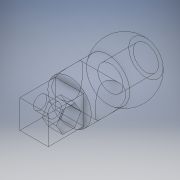
# Autodesk Inventor part: Now as three Part 2
Saved by Autodesk Inventor 2017 (Build 210142000, 142)
## iProperties
Created: 2017-04-12
Part Number: Now as three Part 2
Material: Generic
Document SubType Name: Modeling
Designer: andrew
Density: 1 g/cm^3
Appearance: Default
Author: andrew
Autodesk Inventor part; units mm, degrees
ref_plane "YZ Plane" through (0, 0, 0) normal (1, 0, 0) x (0, 1, 0)
ref_plane "XZ Plane" through (0, 0, 0) normal (0, 1, 0) x (-1, 0, 0)
ref_plane "XY Plane" through (0, 0, 0) normal (0, 0, 1) x (1, 0, 0)
sketch "Sketch1" plane through (0, 0, 0) normal (0, 0, 1) x (1, 0, 0)
  line L0 (0, 6.1628) -> (0, 4.6128)
  line L1 (0, 0) -> (0, -5.3285)
  line L2 (0, -7.6236) -> (0, 6.1628)
  line L3 (7.7918, 0) -> (42.6907, 0)
  line L4 (6.1094, -12.088) -> (6.1094, -4.669)
  line L5 (-6.1094, -10.2236) -> (-6.1094, -4.5067)
  line L6 (0, -7.6236) -> (0, -10.2236)
  line L7 (0, -7.6236) -> (0, -5.0236) construction
  arc A0 (-6.1094, 5.0092) -> (-6.87, -3.5101) centre (0, 0.1701) ccw
  arc A1 (6.1094, -4.669) -> (4.9829, 6.1628) centre (0, 0.1701) ccw
  circle A2 centre (27.3823, 0) radius 1.6
  circle A3 centre (27.3823, 0) radius 1.6
  arc A4 (15.7262, -19.2861) -> (15.9651, 19.4308) centre (0.0053, 0.1701) ccw
  arc A5 (14.9776, -18.1086) -> (14.9776, 18.1086) centre (0, 0) ccw construction
  line L8 (25.0186, 0.0157) -> (19.4598, 0.0157) construction
  line L9 (22.9824, -8.2534) -> (24.1975, 0.0157) construction
  line L10 (24.1975, 0.0157) -> (22.8643, 8.3172) construction
  line L11 (28.9823, 0) -> (30.9823, 0) construction
  line L12 (33.1204, -3.5101) -> (30.9986, 0.1649)
  line L13 (39.4857, -3.5101) -> (33.1204, -3.5101)
  line L14 (39.4857, 0.1649) -> (37.3639, -3.5101)
  circle A6 centre (35.2258, 0) radius 1.9
  line L15 (30.9986, 0.1649) -> (33.1239, 3.846)
  line L16 (33.1239, 3.846) -> (39.4857, 3.8504)
  line L17 (37.3639, 3.8489) -> (39.4857, 0.1649)
  line L18 (39.4857, 0.1784) -> (39.4857, 3.8504)
  line L19 (39.4857, 3.8504) -> (39.4857, -3.5101)
  line L20 (39.4857, 3.8504) -> (39.4857, 5.8504)
  line L21 (39.4857, 5.8504) -> (23.6696, 8.2698)
  arc A7 (15.7262, -19.2861) -> (15.9651, 19.4308) centre (0, 0.1701) ccw
  line L22 (39.4857, -3.5101) -> (39.4857, -5.5101)
  line L23 (39.4857, -5.5101) -> (23.6696, -7.9296)
  line L24 (23.6696, -7.9296) -> (23.6696, 8.2698)
  line L25 (0, 6.1628) -> (0, -10.2236)
  line L26 (0, -12.323) -> (0, -15.7561)
  line L27 (10.9155, -5.0236) -> (17.2808, -5.0236)
  line L28 (17.2808, -8.6986) -> (15.159, -12.3736)
  circle A8 centre (13.0373, -8.6986) radius 1.9
  line L29 (8.7937, -8.6986) -> (10.9155, -5.0236)
  line L30 (17.2808, -12.3736) -> (10.9155, -12.3736)
  line L31 (10.9155, -12.3736) -> (8.7937, -8.6986)
  line L32 (15.159, -5.0236) -> (17.2808, -8.6986)
  line L33 (10.9155, -12.3736) -> (10.9155, -14.3736)
  line L34 (-6.1094, -10.2236) -> (-6.1094, -14.3736)
  line L35 (0, -14.3736) -> (0, -10.2236)
  line L36 (0, -14.3736) -> (0, -19.3736)
  line L37 (-6.1094, -19.3736) -> (-6.1094, -14.3736)
  line L38 (0, -19.3736) -> (0, -25.3736)
  line L39 (0, -25.3736) -> (-6.1094, -25.3736)
  line L40 (-6.1094, -25.3736) -> (-6.1094, -19.3736)
  arc A9 (-4.8255, 6.1628) -> (-6.1094, -4.5067) centre (0, 0.1701) ccw
  line L41 (-5.029, 6.1628) -> (-4.9829, 6.1628)
  line L42 (-4.8255, 6.1628) -> (0, 6.1628)
  dimension "d2" = 3.8
  dimension "d3" = 2
  dimension "d4" = 2
  dimension "d5" = 16
  dimension "d6" = 2
  dimension "d7" = 16
  dimension "d9" = 3.8
  dimension "d10" = 2
  dimension "d17" = 5
  dimension "d50" = 6
  dimension "d64" = 7.7937
  dimension "d65" = 15.388
  constraints: 86 end point, 16 point on circle, 10 centre point, 10 point on line, 6 vertical, 2 collinear, 2 perpendicular, 1 coincident, 1 horizontal, 1 parallel
  measures "d2" diameter of A6
  measures "d3" distance of L11.start L11.end
  measures "d4" distance of L16.end L21.start
  measures "d5" distance of L21.start L21.end
  measures "d6" distance of L19.end L22.end
  measures "d7" distance of L22.end L23.end
  measures "d9" diameter of A8
  measures "d10" distance of L30.end L33.end
  measures "d17" distance of L35.start L36.end
  measures "d50" distance of L36.end L38.end
  measures "d64" radius of A0
  measures "d65" diameter of A9
revolve "Revolution1" add sketch "Sketch1" angle 360 about axis through (0, -12.323, 0) along (0, -1, 0) contours L0 L2 L1 L6 L35 L26 L36 L38 L39 L40 L37 L34 L5 A9 L42
sketch "Sketch2" plane through (0, 0, 0) normal (1, 0, 0) x (0, 1, 0)
  line L0 (-4.669, 0) -> (-6.7907, -3.675) construction
  line L1 (-6.7907, 3.675) -> (-4.669, 0) construction
  line L2 (-15.156, 0) -> (-13.156, 0) construction
  line L3 (-11.0343, -3.675) -> (-6.7907, -3.675) construction
  line L4 (-4.5067, -6.1094) -> (-4.5067, 6.1094) construction
  line L5 (-4.5067, -6.1094) -> (-4.5067, 6.1094) construction
  line L6 (-48.8073, 0) -> (-58.5119, 0) construction
  line L7 (-8.9125, 0) -> (-6.3144, -1.5) construction
  line L8 (-17.8945, -2.9836) -> (-21.3586, -2.9836)
  line L9 (-21.3586, -2.9836) -> (-23.0907, 0.0164)
  line L10 (-23.0907, 0.0164) -> (-21.3586, 3.0164)
  line L11 (-21.3586, 3.0164) -> (-17.8945, 3.0164)
  line L12 (-17.8945, 3.0164) -> (-16.1625, 0.0164)
  line L13 (-16.1625, 0.0164) -> (-17.8945, -2.9836)
  line L14 (23.6533, 6.6124) -> (23.3606, 8.9041) construction
  line L15 (29.9823, 11.5805) -> (34.9823, 11.5805) construction
  line L16 (24.1789, 0) -> (22.8458, 8.3015) construction
  line L17 (25, 0) -> (19.4412, 0) construction
  line L18 (25.1551, -0.0164) -> (29.5051, -0.0164) construction
  line L19 (23.6533, -6.0645) -> (23.6533, 6.6124) construction
  arc A0 (14.9776, -18.1086) -> (14.9776, 18.1086) centre (0, 0) ccw construction
  arc A1 (18.0021, -17.3472) -> (18.0021, 17.3472) centre (0, 0) ccw construction
  arc A2 (18.0021, -17.3472) -> (18.0021, 17.3472) centre (0, 0) ccw construction
  line L20 (22.9638, -8.2692) -> (24.1789, 0) construction
  circle A3 centre (29.5051, -0.0164) radius 4.35 construction
  line L21 (43.4694, -5.828) -> (23.3606, -8.9041) construction
  line L22 (43.4694, 5.828) -> (23.3606, 8.9041) construction
  line L23 (37.4871, -3) -> (35.7551, 0) construction
  line L24 (35.7551, 0) -> (37.4871, 3) construction
  line L25 (43.4694, 5.828) -> (43.4694, -5.828) construction
  circle A4 centre (39.2192, 0) radius 1.9 construction
  line L26 (25, 0) -> (20.4835, 0) construction
  line L27 (23.6533, -6.0645) -> (23.3606, -8.9041) construction
  line L28 (43.4694, 0) -> (43.4694, 5.828) construction
  line L29 (43.4694, -5.828) -> (43.4694, 5.828) construction
  line L30 (29.5346, 0.0703) -> (29.5346, 0.0867) construction
  line L31 (37.4871, 3) -> (43.4694, 3.5234) construction
  line L32 (37.4871, -3) -> (43.4694, -3.5234) construction
  circle A5 centre (-17.0481, 18.2856) radius 1.75
  line L33 (-15.4481, 18.2856) -> (-13.4481, 18.2856) construction
  line L34 (-11.3263, 14.6106) -> (-13.4481, 18.2856) construction
  line L35 (-13.4481, 18.2856) -> (-11.3263, 21.9606) construction
  circle A6 centre (-9.2045, 18.2856) radius 1.9
  line L36 (-4.961, 18.2856) -> (-7.0828, 14.6106) construction
  line L37 (-7.0828, 21.9606) -> (-4.961, 18.2856) construction
  line L38 (-11.3263, 21.9606) -> (-7.0828, 21.9606) construction
  line L39 (-11.3263, 14.6106) -> (-7.0828, 14.6106) construction
  line L40 (-9.2045, 18.2856) -> (-6.6065, 16.7856)
  line L41 (-7.4725, 15.2856) -> (-10.9366, 15.2856)
  line L42 (-10.9366, 15.2856) -> (-12.6686, 18.2856)
  line L43 (-12.6686, 18.2856) -> (-10.9366, 21.2856)
  line L44 (-10.9366, 21.2856) -> (-7.4725, 21.2856)
  line L45 (-7.4725, 21.2856) -> (-5.7404, 18.2856)
  line L46 (-5.7404, 18.2856) -> (-7.4725, 15.2856)
  circle A7 centre (-19.6266, 0.0164) radius 1.9 construction
  circle A8 centre (-9.9125, 0) radius 4.35
  line L47 (-8.9125, 0) -> (-9.9125, 0)
  line L48 (-8.9125, 0) -> (-7.9125, 0) construction
  line L49 (-23.0907, 0.0164) -> (-25.0907, 0.0164)
  point P0 (23.6533, 8.0944)
  point P1 (23.6533, -8.0944)
  point P2 (39.2192, 3)
  point P3 (39.2192, 0)
  point P4 (43.4694, -3)
  point P5 (43.4694, 3)
  dimension "d37" = 3
  dimension "d42" = 3.8
  dimension "d43" = 2
  dimension "d44" = 3.5
  dimension "d45" = 7.35
  dimension "d46" = 3
  dimension "d47" = 1
  dimension "d48" = 180
  dimension "d49" = 2
  constraints: 96 end point, 11 point on circle, 8 centre point, 6 horizontal, 6 point on line, 2 coincident, 1 collinear, 1 horizontal alignment, 1 midpoint, 1 parallel, 1 vertical, 20 other
  measures "d37" distance of L7.start L7.end
  measures "d42" diameter of A6
  measures "d43" distance of L33.start L33.end
  measures "d44" diameter of A5
  measures "d45" distance between parallel lines of L36 L35
  measures "d46" distance of L40.start L40.end
  measures "d47" distance of L47.start L47.end
  measures "d48" angle of L47 L48
  measures "d49" distance of L9.end L49.end
extrude "Extrusion1" cut sketch "Sketch2" along normal blind 10 contours L8 L9 L10 L11 L12 L13 | A8
sketch "Sketch4" plane through (0, 0, 0) normal (1, 0, 0) x (0, 0, -1)
  line L0 (0, -15.156) -> (0, -13.156) construction
  line L1 (0, -4.669) -> (3.675, -6.7907) construction
  line L2 (-3.675, -6.7907) -> (0, -4.669) construction
  line L3 (3.675, -11.0343) -> (3.675, -6.7907) construction
  line L4 (6.1094, -4.669) -> (-6.1094, -4.669) construction
  line L5 (6.1094, -4.669) -> (-6.1094, -4.669) construction
  line L6 (0, -8.9125) -> (1.5, -6.3144) construction
  line L7 (2.9836, -17.8945) -> (2.9836, -21.3586)
  line L8 (2.9836, -21.3586) -> (-0.0164, -23.0907)
  line L9 (-0.0164, -23.0907) -> (-3.0164, -21.3586)
  line L10 (-3.0164, -21.3586) -> (-3.0164, -17.8945)
  line L11 (-3.0164, -17.8945) -> (-0.0164, -16.1625)
  line L12 (-0.0164, -16.1625) -> (2.9836, -17.8945)
  circle A0 centre (-0.0164, -19.6266) radius 1.9
  circle A1 centre (0, -9.9125) radius 4.35
  line L13 (0, -8.9125) -> (0, -9.9125)
  line L14 (0, -8.9125) -> (0, -7.9125) construction
  line L15 (-0.0164, -23.0907) -> (-0.0164, -25.0907)
  point P0 (0, -4.669)
  point P1 (6.1094, -4.669)
  point P2 (-6.1094, -4.669)
  point P3 (-0.0164, -23.0907)
  dimension "d51" = 3
  dimension "d52" = 1
  dimension "d53" = 180
  dimension "d54" = 2
  constraints: 32 end point, 2 centre point, 1 coincident, 1 collinear
  measures "d51" distance of L6.start L6.end
  measures "d52" distance of L13.start L13.end
  measures "d53" angle of L13 L14
  measures "d54" distance of L8.end L15.end
extrude "Extrusion2" cut sketch "Sketch4" against normal blind 10 and the other way blind 5 contours A0 | A1
sketch "Sketch7" plane through (0, -25.3736, 0) normal (0, -1, 0) x (1, 0, 0)
  line L0 (0, 0.0164) -> (6.1094, 0.0164) construction
  line L1 (0, 0.0164) -> (-4, 0.0164) construction
  line L2 (-4, 0.0164) -> (-4, 4.0164) construction
  line L3 (-4, 4.0164) -> (0, 4.0164) construction
  line L4 (0, 4.0164) -> (0, 0.0164) construction
  line L5 (-4, 4.0164) -> (4, 4.0164)
  line L6 (4, 4.0164) -> (4, -3.9836)
  line L7 (4, -3.9836) -> (-4, -3.9836)
  line L8 (-4, -3.9836) -> (-4, 4.0164)
  line L9 (-4, -9.4779) -> (-8.9104, -9.4779)
  line L10 (-8.9104, -9.4779) -> (-8.9104, 10.8185)
  line L11 (-8.9104, 10.8185) -> (-4, 10.8185)
  line L12 (-4, 10.8185) -> (-4, -9.4779)
  line L13 (-7.8642, 4.0164) -> (7.4627, 4.0164)
  line L14 (7.4627, 4.0164) -> (7.4627, 9.8769)
  line L15 (7.4627, 9.8769) -> (-7.8642, 9.8769)
  line L16 (-7.8642, 9.8769) -> (-7.8642, 4.0164)
  line L17 (4, -8.5624) -> (10.7059, -8.5624)
  line L18 (10.7059, -8.5624) -> (10.7059, 4.0164)
  line L19 (10.7059, 4.0164) -> (4, 4.0164)
  line L20 (4, 4.0164) -> (4, -8.5624)
  line L21 (4, -12.198) -> (-4, -12.198)
  line L22 (-4, -12.198) -> (-4, -3.9836)
  line L23 (-4, -3.9836) -> (4, -3.9836)
  line L24 (4, -3.9836) -> (4, -12.198)
  dimension "d70" = 4
  dimension "d71" = 4
  dimension "d72" = 8
  dimension "d73" = 8
  constraints: 48 end point, 12 parallel, 6 horizontal, 6 perpendicular, 2 point on line
  measures "d70" distance of L2.end L3.end
  measures "d71" distance of L1.end L2.end
  measures "d72" distance of L6.end L7.end
  measures "d73" distance of L5.end L6.end
extrude "Extrusion5" cut sketch "Sketch7" against normal blind 10 contours L12 L15 L14 L13 L5 | L13 L16 L15 L12 | L8 L12 L9 L10 L11 L15 L16 L13 | L13 L19 L18 L17 L20 L6 | L7 L20 L24 L21 L22 L12
sketch "Sketch8" plane through (0, 6.1628, 0) normal (0, 1, 0) x (1, 0, 0)
  circle A0 centre (0, 0) radius 3.56
  dimension "d66" = 7.12
  constraints: 1 centre point, 1 coincident
  measures "d66" diameter of A0
extrude "Extrusion6" cut sketch "Sketch8" against normal blind 10
body "Solid1"
